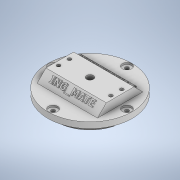
# Autodesk Inventor part: Union_rotatoria_lazy_susan
Saved by Autodesk Inventor 2021 (Build 250183000, 183)
## iProperties
Created: 2021-01-16
Part Number: Union_rotatoria_lazy_susan
Material: Generic
Document SubType Name: Modeling
Designer: jorge
Density: 1 g/cm^3
Appearance: Default
Author: jorge
Autodesk Inventor part; units mm, degrees
ref_plane "YZ Plane" through (0, 0, 0) normal (1, 0, 0) x (0, 1, 0)
ref_plane "XZ Plane" through (0, 0, 0) normal (0, 1, 0) x (-1, 0, 0)
ref_plane "XY Plane" through (0, 0, 0) normal (0, 0, 1) x (1, 0, 0)
sketch "Sketch1" plane through (0, 0, 0) normal (0, 1, 0) x (-1, 0, 0)
  circle A0 centre (0, 0) radius 50
  circle A1 centre (0, 0) radius 4.05
  circle A2 centre (0, 44) radius 2.25
  circle A3 centre (44, 0) radius 2.25
  circle A4 centre (0, -44) radius 2.25
  circle A5 centre (-44, 0) radius 2.25
  dimension "d0" = 100
  dimension "d1" = 8.1
  dimension "d2" = 4.5
  dimension "d3" = 4.5
  dimension "d4" = 4.5
  dimension "d5" = 4.5
  dimension "d6" = 88
  dimension "d7" = 88
  dimension "d8" = 0
  dimension "d9" = 0
  dimension "d10" = 0
  dimension "d11" = 0
  dimension "d12" = 44
  dimension "d13" = 44
  constraints: 6 centre point, 2 coincident
  measures "d0" diameter of A0
  measures "d1" diameter of A1
  measures "d2" diameter of A2
  measures "d3" diameter of A3
  measures "d4" diameter of A4
  measures "d5" diameter of A5
  measures "d6" distance of A4.centre A2.centre
  measures "d7" distance of A5.centre A3.centre
  measures "d8" vertical distance of point (0, 0) A3.centre
  measures "d9" vertical distance of A5.centre point (0, 0)
  measures "d10" horizontal distance of A2.centre point (0, 0)
  measures "d11" horizontal distance of A4.centre point (0, 0)
  measures "d12" distance of A4.centre point (0, 0)
  measures "d13" distance of point (0, 0) A3.centre
extrude "Extrusion1" add sketch "Sketch1" along normal blind 7
sketch "Sketch2" plane through (0, 0, 0) normal (0, -1, 0) x (1, 0, 0)
  circle A0 centre (0, 0) radius 4.05
  circle A1 centre (0, 0) radius 4.05 projected
  circle A2 centre (0, 0) radius 39.9
  dimension "d16" = 79.8
  constraints: 2 centre point, 2 coincident, 1 concentric
  measures "d16" diameter of A2
extrude "Extrusion2" add sketch "Sketch2" along normal blind 8.5
sketch "Sketch7" plane through (0, -8.5, 0) normal (0, -1, 0) x (1, 0, 0)
  circle A0 centre (0, 0) radius 4.05 projected
  circle A1 centre (0, 0) radius 12.75
  circle A2 centre (0, 0) radius 39.9 projected
  circle A3 centre (0, 0) radius 4.05 projected
  line L0 (4.05, 4.05) -> (-4.05, 4.05)
  line L1 (-4.05, 4.05) -> (-4.05, -39.9)
  line L2 (-4.05, -39.9) -> (4.05, -39.9)
  line L3 (4.05, -39.9) -> (4.05, 4.05)
  line L4 (39.9, -4.05) -> (-4.05, -4.05)
  line L5 (-4.05, -4.05) -> (-4.05, 4.05)
  line L6 (-4.05, 4.05) -> (39.9, 4.05)
  line L7 (39.9, 4.05) -> (39.9, -4.05)
  point P0 (39.6939, 4.05)
  point P1 (12.0897, 4.05)
  point P2 (12.0897, -4.05)
  point P3 (39.6939, -4.05)
  point P4 (4.05, -39.6939)
  point P5 (4.05, -12.0897)
  point P6 (-4.05, -12.0897)
  point P7 (-4.05, -39.6939)
  dimension "d30" = 25.5
  constraints: 16 end point, 8 tangent, 4 parallel, 2 horizontal, 2 perpendicular, 1 centre point, 1 coincident
  measures "d30" diameter of A1
extrude "Extrusion7" cut sketch "Sketch7" against normal blind 6 contours A0 | L3 L4 A0 | A0 L0 L3 | L3 L6 A1 L4 | L0 L1 A1 L6 | A0 L1 L0 | L4 L1 A0 | L4 L3 A1 L1 | L4 A1 L3 | L6 A2 L4 A1 | L3 A2 L1 A1
chamfer "Chamfer1" distance 6 angle 45 4 edges at (-4.05, -8.5, -25.8918) (4.05, -8.5, -25.8918) (25.8918, -8.5, -4.05) (25.8918, -8.5, 4.05)
sketch "Sketch11" plane through (0, 7, 0) normal (0, 1, 0) x (1, 0, 0)
  circle A0 centre (0, 0) radius 4.05 projected
  circle A1 centre (0, 0) radius 4.05
  line L0 (-35.9605, -16.5) -> (35.9605, -16.5)
  line L1 (35.9605, -16.5) -> (35.9605, 16.5)
  line L2 (35.9605, 16.5) -> (-35.9605, 16.5)
  line L3 (-35.9605, 16.5) -> (-35.9605, -16.5)
  circle A2 centre (-30.9605, -6.5) radius 2.1
  circle A3 centre (31.2395, -6.5) radius 2.1
  circle A4 centre (31.2395, 6.5) radius 2.1
  circle A5 centre (-30.9605, 6.5) radius 2.1
  dimension "d39" = 71.921
  dimension "d40" = 33
  dimension "d41" = 35.9605
  dimension "d42" = 16.5
  dimension "d43" = 4.2
  dimension "d44" = 4.2
  dimension "d45" = 4.2
  dimension "d46" = 4.2
  dimension "d47" = 13
  dimension "d48" = 13
  dimension "d49" = 62.2
  dimension "d50" = 62.2
  dimension "d51" = 5
  dimension "d52" = 10
  dimension "d53" = 10
  dimension "d54" = 10
  constraints: 8 end point, 5 centre point, 2 parallel, 1 coincident, 1 concentric, 1 horizontal, 1 perpendicular
  measures "d39" distance between parallel lines of L1 L3
  measures "d40" distance between parallel lines of L2 L0
  measures "d41" distance from line of point (0, 0) L3
  measures "d42" distance from line of L2 point (0, 0)
  measures "d43" diameter of A2
  measures "d44" diameter of A3
  measures "d45" diameter of A4
  measures "d46" diameter of A5
  measures "d47" distance of A5.centre A2.centre
  measures "d48" distance of A4.centre A3.centre
  measures "d49" distance of A4.centre A5.centre
  measures "d50" distance of A3.centre A2.centre
  measures "d51" distance from line of A2.centre L3
  measures "d52" distance from line of L0 A2.centre
  measures "d53" distance from line of L0 A3.centre
  measures "d54" distance from line of L2 A5.centre
extrude "Extrusion9" add sketch "Sketch11" along normal blind 10.5
chamfer "Chamfer2" distance 10.5 angle 45 2 edges at (0, 7, -16.5) (0, 7, 16.5)
sketch "Sketch12" plane through (0, 17.5, 0) normal (0, 1, 0) x (1, 0, 0)
  circle A0 centre (-30.9605, -6.5) radius 2.1 projected
  circle A1 centre (-30.9605, -6.5) radius 2.1
  circle A2 centre (-30.9605, 6.5) radius 2.1 projected
  circle A3 centre (-30.9605, 6.5) radius 2.1
  circle A4 centre (31.2395, -6.5) radius 2.1 projected
  circle A5 centre (31.2395, -6.5) radius 2.1
  circle A6 centre (31.2395, 6.5) radius 2.1 projected
  circle A7 centre (31.2395, 6.5) radius 2.1
  point P0 (0, 0)
  constraints: 4 centre point, 4 coincident, 4 concentric
extrude "Extrusion10" cut sketch "Sketch12" against normal up to surface (26 mm away)
sketch "Sketch13" plane through (0, -8.5, 0) normal (0, -1, 0) x (1, 0, 0)
  circle A0 centre (31.2395, -6.5) radius 2.1 projected
  line L0 (29.2188, -10) -> (27.198, -6.5)
  line L1 (27.198, -6.5) -> (29.2188, -3)
  line L2 (29.2188, -3) -> (33.2602, -3)
  line L3 (33.2602, -3) -> (35.281, -6.5)
  line L4 (35.281, -6.5) -> (33.2602, -10)
  line L5 (33.2602, -10) -> (29.2188, -10)
  circle A1 centre (31.2395, 6.5) radius 2.1 projected
  line L6 (29.2188, 10) -> (33.2602, 10)
  line L7 (33.2602, 10) -> (35.281, 6.5)
  line L8 (35.281, 6.5) -> (33.2602, 3)
  line L9 (33.2602, 3) -> (29.2188, 3)
  line L10 (29.2188, 3) -> (27.198, 6.5)
  line L11 (27.198, 6.5) -> (29.2188, 10)
  circle A2 centre (-30.9605, 6.5) radius 2.1 projected
  line L12 (-28.9398, 3) -> (-32.9812, 3)
  line L13 (-32.9812, 3) -> (-35.002, 6.5)
  line L14 (-35.002, 6.5) -> (-32.9812, 10)
  line L15 (-32.9812, 10) -> (-28.9398, 10)
  line L16 (-28.9398, 10) -> (-26.919, 6.5)
  line L17 (-26.919, 6.5) -> (-28.9398, 3)
  circle A3 centre (-30.9605, -6.5) radius 2.1 projected
  line L18 (-28.9398, -10) -> (-32.9812, -10)
  line L19 (-32.9812, -10) -> (-35.002, -6.5)
  line L20 (-35.002, -6.5) -> (-32.9812, -3)
  line L21 (-32.9812, -3) -> (-28.9398, -3)
  line L22 (-28.9398, -3) -> (-26.919, -6.5)
  line L23 (-26.919, -6.5) -> (-28.9398, -10)
  point P0 (0, 0)
  dimension "d62" = 7
  dimension "d63" = 7
  dimension "d64" = 7
  dimension "d65" = 7
  constraints: 48 end point, 4 coincident, 2 collinear, 52 other
  measures "d62" distance between parallel lines of L2 L5
  measures "d63" distance between parallel lines of L6 L9
  measures "d64" distance between parallel lines of L21 L18
  measures "d65" distance between parallel lines of L16 L13
extrude "Extrusion11" cut sketch "Sketch13" against normal blind 10 contours A0 | L0 L1 L2 L3 L4 L5 | A1 | L6 L7 L8 L9 L10 L11 | A2 | L12 L13 L14 L15 L16 L17 | A3 | L18 L19 L20 L21 L22 L23
chamfer "Chamfer3" distance 2 angle 45 12 edges at (-27.9294, -8.5, -8.25) (-27.9294, -8.5, -4.75) (-30.9605, -8.5, -3) (-33.9916, -8.5, -4.75) (-33.9916, -8.5, -8.25) (-30.9605, -8.5, -10) (-27.9294, -8.5, 8.25) (-27.9294, -8.5, 4.75) (-30.9605, -8.5, 3) (-33.9916, -8.5, 4.75) (-33.9916, -8.5, 8.25) (-30.9605, -8.5, 10)
sketch "Sketch14" plane through (0, 7, 0) normal (0, 1, 0) x (1, 0, 0)
  circle A0 centre (0, 44) radius 2.25 projected
  circle A1 centre (0, 44) radius 5.5
  circle A2 centre (44, 0) radius 2.25 projected
  circle A3 centre (44, 0) radius 5.5
  circle A4 centre (-44, 0) radius 2.25 projected
  circle A5 centre (-44, 0) radius 5.5
  circle A6 centre (0, -44) radius 2.25 projected
  circle A7 centre (0, -44) radius 5.5
  point P0 (0, 0)
  dimension "d71" = 11
  dimension "d72" = 11
  dimension "d73" = 11
  dimension "d74" = 11
  constraints: 4 centre point, 4 coincident
  measures "d71" diameter of A1
  measures "d72" diameter of A3
  measures "d73" diameter of A5
  measures "d74" diameter of A7
extrude "Extrusion12" cut sketch "Sketch14" against normal blind 2 contours A0 | A1 | A2 | A3 | A4 | A5 | A6 | A7
sketch "Sketch15" plane through (-35.9605, 17.5, 16.5) normal (0, 0.7071068, 0.7071068) x (1, 0, 0)
  line L0 (10.3561, -2.2132) -> (62.4016, -2.2132) construction
  line L1 (62.4016, -2.2132) -> (62.4016, -11.2501) construction
  line L2 (62.4016, -11.2501) -> (10.3561, -11.2501) construction
  line L3 (10.3561, -11.2501) -> (10.3561, -2.2132) construction
  line L4 (14.5652, -9.3494) -> (10.7986, -9.3494)
  line L5 (10.7986, -9.3494) -> (10.7986, -8.1298)
  line L6 (10.7986, -8.1298) -> (11.8026, -8.1298)
  line L7 (11.8026, -8.1298) -> (11.8026, -3.569)
  line L8 (11.8026, -3.569) -> (10.7986, -3.569)
  line L9 (10.7986, -3.569) -> (10.7986, -2.3494)
  line L10 (10.7986, -2.3494) -> (14.5652, -2.3494)
  line L11 (14.5652, -2.3494) -> (14.5652, -3.569)
  line L12 (14.5652, -3.569) -> (13.5612, -3.569)
  line L13 (13.5612, -3.569) -> (13.5612, -8.1298)
  line L14 (13.5612, -8.1298) -> (14.5652, -8.1298)
  line L15 (14.5652, -8.1298) -> (14.5652, -9.3494)
  line L16 (21.7297, -9.3494) -> (20.0393, -9.3494)
  line L17 (20.0393, -9.3494) -> (17.3391, -4.4709)
  line L18 (17.3391, -4.4709) -> (17.3391, -9.3494)
  line L19 (17.3391, -9.3494) -> (15.7338, -9.3494)
  line L20 (15.7338, -9.3494) -> (15.7338, -2.3494)
  line L21 (15.7338, -2.3494) -> (17.8894, -2.3494)
  line L22 (17.8894, -2.3494) -> (20.1244, -6.3599)
  line L23 (20.1244, -6.3599) -> (20.1244, -2.3494)
  line L24 (20.1244, -2.3494) -> (21.7297, -2.3494)
  line L25 (21.7297, -2.3494) -> (21.7297, -9.3494)
  spline S0 degree 2 poles (28.9963, -8.9523) (28.5368, -9.1395) (27.0676, -9.4969) (26.3529, -9.4969) knots 0 0 0 1 2 2 2
  spline S1 degree 2 poles (26.3529, -9.4969) (24.7022, -9.4969) (22.7451, -7.5909) (22.7451, -5.8437) knots 0 0 0 1 2 2 2
  spline S2 degree 2 poles (22.7451, -5.8437) (22.7451, -4.1987) (24.7022, -2.2132) (26.4039, -2.2132) knots 0 0 0 1 2 2 2
  spline S3 degree 2 poles (26.4039, -2.2132) (27.2832, -2.2132) (28.3837, -2.5479) (28.968, -2.8316) knots 0 0 0 1 2 2 2
  line L26 (28.968, -2.8316) -> (28.968, -4.4766)
  line L27 (28.968, -4.4766) -> (28.8091, -4.4766)
  spline S4 degree 2 poles (28.8091, -4.4766) (28.6843, -4.3802) (28.2078, -4.0115) (27.9809, -3.8867) knots 0 0 0 1 2 2 2
  spline S5 degree 2 poles (27.9809, -3.8867) (27.72, -3.7335) (27.0279, -3.5179) (26.6422, -3.5179) knots 0 0 0 1 2 2 2
  spline S6 degree 2 poles (26.6422, -3.5179) (26.1941, -3.5179) (25.4509, -3.8016) (25.1616, -4.0909) knots 0 0 0 1 2 2 2
  spline S7 degree 2 poles (25.1616, -4.0909) (24.8837, -4.3745) (24.5603, -5.2424) (24.5603, -5.8154) knots 0 0 0 1 2 2 2
  spline S8 degree 2 poles (24.5603, -5.8154) (24.5603, -7.0406) (25.7913, -8.2092) (26.8521, -8.2092) knots 0 0 0 1 2 2 2
  spline S9 degree 2 poles (26.8521, -8.2092) (26.9485, -8.2092) (27.1981, -8.1978) (27.2945, -8.1922) knots 0 0 0 1 2 2 2
  line L28 (27.2945, -8.1922) -> (27.2945, -6.8137)
  line L29 (27.2945, -6.8137) -> (25.9388, -6.8137)
  line L30 (25.9388, -6.8137) -> (25.9388, -5.5034)
  line L31 (25.9388, -5.5034) -> (28.9963, -5.5034)
  line L32 (28.9963, -5.5034) -> (28.9963, -8.9523)
  line L33 (35.8035, -10.9718) -> (29.5239, -10.9718)
  line L34 (29.5239, -10.9718) -> (29.5239, -10.0244)
  line L35 (29.5239, -10.0244) -> (35.8035, -10.0244)
  line L36 (35.8035, -10.0244) -> (35.8035, -10.9718)
  line L37 (43.6033, -9.3494) -> (41.8561, -9.3494)
  line L38 (41.8561, -9.3494) -> (41.8561, -4.7092)
  line L39 (41.8561, -4.7092) -> (40.5855, -7.7043)
  line L40 (40.5855, -7.7043) -> (39.3829, -7.7043)
  line L41 (39.3829, -7.7043) -> (38.1122, -4.7092)
  line L42 (38.1122, -4.7092) -> (38.1122, -9.3494)
  line L43 (38.1122, -9.3494) -> (36.4558, -9.3494)
  line L44 (36.4558, -9.3494) -> (36.4558, -2.3494)
  line L45 (36.4558, -2.3494) -> (38.4809, -2.3494)
  line L46 (38.4809, -2.3494) -> (40.0352, -5.804)
  line L47 (40.0352, -5.804) -> (41.5782, -2.3494)
  line L48 (41.5782, -2.3494) -> (43.6033, -2.3494)
  line L49 (43.6033, -2.3494) -> (43.6033, -9.3494)
  line L50 (44.301, -9.3494) -> (46.6665, -2.3494)
  line L51 (46.6665, -2.3494) -> (48.5838, -2.3494)
  line L52 (48.5838, -2.3494) -> (50.9493, -9.3494)
  line L53 (50.9493, -9.3494) -> (49.1398, -9.3494)
  line L54 (49.1398, -9.3494) -> (48.703, -7.9199)
  line L55 (48.703, -7.9199) -> (46.502, -7.9199)
  line L56 (46.502, -7.9199) -> (46.0595, -9.3494)
  line L57 (46.0595, -9.3494) -> (44.301, -9.3494)
  line L58 (48.3172, -6.6492) -> (47.6025, -4.3348)
  line L59 (47.6025, -4.3348) -> (46.8821, -6.6492)
  line L60 (46.8821, -6.6492) -> (48.3172, -6.6492)
  line L61 (52.9915, -9.3494) -> (52.9915, -3.6825)
  line L62 (52.9915, -3.6825) -> (50.921, -3.6825)
  line L63 (50.921, -3.6825) -> (50.921, -2.3494)
  line L64 (50.921, -2.3494) -> (56.8205, -2.3494)
  line L65 (56.8205, -2.3494) -> (56.8205, -3.6825)
  line L66 (56.8205, -3.6825) -> (54.75, -3.6825)
  line L67 (54.75, -3.6825) -> (54.75, -9.3494)
  line L68 (54.75, -9.3494) -> (52.9915, -9.3494)
  line L69 (57.5409, -9.3494) -> (57.5409, -2.3494)
  line L70 (57.5409, -2.3494) -> (62.2719, -2.3494)
  line L71 (62.2719, -2.3494) -> (62.2719, -3.6825)
  line L72 (62.2719, -3.6825) -> (59.2881, -3.6825)
  line L73 (59.2881, -3.6825) -> (59.2881, -4.9134)
  line L74 (59.2881, -4.9134) -> (62.0393, -4.9134)
  line L75 (62.0393, -4.9134) -> (62.0393, -6.2465)
  line L76 (62.0393, -6.2465) -> (59.2881, -6.2465)
  line L77 (59.2881, -6.2465) -> (59.2881, -8.0163)
  line L78 (59.2881, -8.0163) -> (62.2719, -8.0163)
  line L79 (62.2719, -8.0163) -> (62.2719, -9.3494)
  line L80 (62.2719, -9.3494) -> (57.5409, -9.3494)
  point P0 (35.9605, -0.7071)
  constraints: 2 other
extrude "Extrusion13" add sketch "Sketch15" along normal blind 1.5
sketch "Sketch16" plane through (35.9605, 17.5, -16.5) normal (0, 0.7071068, -0.7071068) x (-1, 0, 0)
  line L0 (4.2099, -2.9037) -> (67.9107, -2.9037) construction
  line L1 (67.9107, -2.9037) -> (67.9107, -13.0878) construction
  line L2 (67.9107, -13.0878) -> (4.2099, -13.0878) construction
  line L3 (4.2099, -13.0878) -> (4.2099, -2.9037) construction
  spline S0 degree 2 poles (7.0973, -10.3405) (6.2918, -10.3405) (5.0778, -10.0285) (4.556, -9.8016) knots 0 0 0 1 2 2 2
  line L4 (4.556, -9.8016) -> (4.556, -8.1338)
  line L5 (4.556, -8.1338) -> (4.7148, -8.1338)
  spline S1 degree 2 poles (4.7148, -8.1338) (5.2424, -8.582) (6.5073, -9.0641) (7.103, -9.0641) knots 0 0 0 1 2 2 2
  spline S2 degree 2 poles (7.103, -9.0641) (7.2561, -9.0641) (7.7496, -8.9961) (7.8971, -8.928) knots 0 0 0 1 2 2 2
  spline S3 degree 2 poles (7.8971, -8.928) (8.0787, -8.8486) (8.3339, -8.5593) (8.3339, -8.3267) knots 0 0 0 1 2 2 2
  spline S4 degree 2 poles (8.3339, -8.3267) (8.3339, -8.0601) (7.9198, -7.7311) (7.6362, -7.6573) knots 0 0 0 1 2 2 2
  spline S5 degree 2 poles (7.6362, -7.6573) (7.2788, -7.5609) (6.4676, -7.3964) (6.1103, -7.2716) knots 0 0 0 1 2 2 2
  spline S6 degree 2 poles (6.1103, -7.2716) (5.2991, -6.988) (4.5957, -6.0179) (4.5957, -5.2919) knots 0 0 0 1 2 2 2
  spline S7 degree 2 poles (4.5957, -5.2919) (4.5957, -4.3105) (6.2578, -3.0909) (7.5057, -3.0909) knots 0 0 0 1 2 2 2
  spline S8 degree 2 poles (7.5057, -3.0909) (8.1297, -3.0909) (9.3663, -3.3462) (9.8542, -3.5617) knots 0 0 0 1 2 2 2
  line L6 (9.8542, -3.5617) -> (9.8542, -5.1614)
  line L7 (9.8542, -5.1614) -> (9.701, -5.1614)
  spline S9 degree 2 poles (9.701, -5.1614) (9.3096, -4.8267) (8.1864, -4.3672) (7.5965, -4.3672) knots 0 0 0 1 2 2 2
  spline S10 degree 2 poles (7.5965, -4.3672) (7.3639, -4.3672) (7.0009, -4.4353) (6.7966, -4.5261) knots 0 0 0 1 2 2 2
  spline S11 degree 2 poles (6.7966, -4.5261) (6.6321, -4.5998) (6.3939, -4.8948) (6.3939, -5.0763) knots 0 0 0 1 2 2 2
  spline S12 degree 2 poles (6.3939, -5.0763) (6.3939, -5.3486) (6.774, -5.6606) (7.3185, -5.7854) knots 0 0 0 1 2 2 2
  spline S13 degree 2 poles (7.3185, -5.7854) (7.6702, -5.8648) (8.3226, -6.0179) (8.697, -6.1484) knots 0 0 0 1 2 2 2
  spline S14 degree 2 poles (8.697, -6.1484) (9.4231, -6.415) (10.1321, -7.3) (10.1321, -8.0261) knots 0 0 0 1 2 2 2
  spline S15 degree 2 poles (10.1321, -8.0261) (10.1321, -9.0698) (8.4928, -10.3405) (7.0973, -10.3405) knots 0 0 0 1 2 2 2
  line L8 (14.5171, -10.2157) -> (10.7505, -10.2157)
  line L9 (10.7505, -10.2157) -> (10.7505, -8.9961)
  line L10 (10.7505, -8.9961) -> (11.7545, -8.9961)
  line L11 (11.7545, -8.9961) -> (11.7545, -4.4353)
  line L12 (11.7545, -4.4353) -> (10.7505, -4.4353)
  line L13 (10.7505, -4.4353) -> (10.7505, -3.2157)
  line L14 (10.7505, -3.2157) -> (14.5171, -3.2157)
  line L15 (14.5171, -3.2157) -> (14.5171, -4.4353)
  line L16 (14.5171, -4.4353) -> (13.513, -4.4353)
  line L17 (13.513, -4.4353) -> (13.513, -8.9961)
  line L18 (13.513, -8.9961) -> (14.5171, -8.9961)
  line L19 (14.5171, -8.9961) -> (14.5171, -10.2157)
  line L20 (14.9312, -10.2157) -> (17.2966, -3.2157)
  line L21 (17.2966, -3.2157) -> (19.214, -3.2157)
  line L22 (19.214, -3.2157) -> (21.5795, -10.2157)
  line L23 (21.5795, -10.2157) -> (19.7699, -10.2157)
  line L24 (19.7699, -10.2157) -> (19.3331, -8.7862)
  line L25 (19.3331, -8.7862) -> (17.1321, -8.7862)
  line L26 (17.1321, -8.7862) -> (16.6897, -10.2157)
  line L27 (16.6897, -10.2157) -> (14.9312, -10.2157)
  line L28 (18.9474, -7.5155) -> (18.2326, -5.2011)
  line L29 (18.2326, -5.2011) -> (17.5122, -7.5155)
  line L30 (17.5122, -7.5155) -> (18.9474, -7.5155)
  line L31 (21.5227, -10.2157) -> (23.8882, -3.2157)
  line L32 (23.8882, -3.2157) -> (25.8056, -3.2157)
  line L33 (25.8056, -3.2157) -> (28.171, -10.2157)
  line L34 (28.171, -10.2157) -> (26.3615, -10.2157)
  line L35 (26.3615, -10.2157) -> (25.9247, -8.7862)
  line L36 (25.9247, -8.7862) -> (23.7237, -8.7862)
  line L37 (23.7237, -8.7862) -> (23.2813, -10.2157)
  line L38 (23.2813, -10.2157) -> (21.5227, -10.2157)
  line L39 (25.539, -7.5155) -> (24.8242, -5.2011)
  line L40 (24.8242, -5.2011) -> (24.1038, -7.5155)
  line L41 (24.1038, -7.5155) -> (25.539, -7.5155)
  line L42 (34.8647, -10.2157) -> (33.1743, -10.2157)
  line L43 (33.1743, -10.2157) -> (30.4741, -5.3372)
  line L44 (30.4741, -5.3372) -> (30.4741, -10.2157)
  line L45 (30.4741, -10.2157) -> (28.8688, -10.2157)
  line L46 (28.8688, -10.2157) -> (28.8688, -3.2157)
  line L47 (28.8688, -3.2157) -> (31.0244, -3.2157)
  line L48 (31.0244, -3.2157) -> (33.2594, -7.2262)
  line L49 (33.2594, -7.2262) -> (33.2594, -3.2157)
  line L50 (33.2594, -3.2157) -> (34.8647, -3.2157)
  line L51 (34.8647, -3.2157) -> (34.8647, -10.2157)
  line L52 (45.2399, -10.2157) -> (43.1127, -10.2157)
  line L53 (43.1127, -10.2157) -> (41.2124, -7.3737)
  line L54 (41.2124, -7.3737) -> (40.8663, -7.8502)
  line L55 (40.8663, -7.8502) -> (40.8663, -10.2157)
  line L56 (40.8663, -10.2157) -> (39.1078, -10.2157)
  line L57 (39.1078, -10.2157) -> (39.1078, -3.2157)
  line L58 (39.1078, -3.2157) -> (40.8663, -3.2157)
  line L59 (40.8663, -3.2157) -> (40.8663, -6.3413)
  line L60 (40.8663, -6.3413) -> (43.1127, -3.2157)
  line L61 (43.1127, -3.2157) -> (45.1378, -3.2157)
  line L62 (45.1378, -3.2157) -> (42.6419, -6.4661)
  line L63 (42.6419, -6.4661) -> (45.2399, -10.2157)
  line L64 (45.0584, -10.2157) -> (47.4239, -3.2157)
  line L65 (47.4239, -3.2157) -> (49.3412, -3.2157)
  line L66 (49.3412, -3.2157) -> (51.7067, -10.2157)
  line L67 (51.7067, -10.2157) -> (49.8971, -10.2157)
  line L68 (49.8971, -10.2157) -> (49.4603, -8.7862)
  line L69 (49.4603, -8.7862) -> (47.2594, -8.7862)
  line L70 (47.2594, -8.7862) -> (46.8169, -10.2157)
  line L71 (46.8169, -10.2157) -> (45.0584, -10.2157)
  line L72 (49.0746, -7.5155) -> (48.3599, -5.2011)
  line L73 (48.3599, -5.2011) -> (47.6394, -7.5155)
  line L74 (47.6394, -7.5155) -> (49.0746, -7.5155)
  line L75 (53.7715, -2.9037) -> (53.4879, -5.6719)
  line L76 (53.4879, -5.6719) -> (52.5236, -5.6719)
  line L77 (52.5236, -5.6719) -> (52.2399, -2.9037)
  line L78 (52.2399, -2.9037) -> (53.7715, -2.9037)
  line L79 (54.2991, -10.2157) -> (56.6646, -3.2157)
  line L80 (56.6646, -3.2157) -> (58.5819, -3.2157)
  line L81 (58.5819, -3.2157) -> (60.9474, -10.2157)
  line L82 (60.9474, -10.2157) -> (59.1378, -10.2157)
  line L83 (59.1378, -10.2157) -> (58.701, -8.7862)
  line L84 (58.701, -8.7862) -> (56.5001, -8.7862)
  line L85 (56.5001, -8.7862) -> (56.0576, -10.2157)
  line L86 (56.0576, -10.2157) -> (54.2991, -10.2157)
  line L87 (58.3153, -7.5155) -> (57.6005, -5.2011)
  line L88 (57.6005, -5.2011) -> (56.8801, -7.5155)
  line L89 (56.8801, -7.5155) -> (58.3153, -7.5155)
  line L90 (67.6411, -10.2157) -> (65.9506, -10.2157)
  line L91 (65.9506, -10.2157) -> (63.2505, -5.3372)
  line L92 (63.2505, -5.3372) -> (63.2505, -10.2157)
  line L93 (63.2505, -10.2157) -> (61.6451, -10.2157)
  line L94 (61.6451, -10.2157) -> (61.6451, -3.2157)
  line L95 (61.6451, -3.2157) -> (63.8007, -3.2157)
  line L96 (63.8007, -3.2157) -> (66.0357, -7.2262)
  line L97 (66.0357, -7.2262) -> (66.0357, -3.2157)
  line L98 (66.0357, -3.2157) -> (67.6411, -3.2157)
  line L99 (67.6411, -3.2157) -> (67.6411, -10.2157)
  point P0 (35.9605, -0.7071)
  constraints: 2 other
extrude "Extrusion14" add sketch "Sketch16" along normal blind 1.5
body "Solid1"
